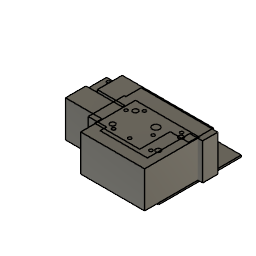
Valve mount (Autodesk Fusion 360 design; units mm, degrees)
Autodesk Fusion 360 part; units mm, degrees
sketch "Sketch3" plane through (0, 0, 0) normal (0, 0, 1) x (1, 0, 0)
  circle A0 centre (-19.4392, 58.0614) radius 3.5
  circle A1 centre (62.5608, 58.0614) radius 3.5
  circle A2 centre (-19.4392, -9.4386) radius 3.5
  circle A3 centre (62.5608, -9.4386) radius 3.5
  line L0 (-30, 76.3146) -> (73.519, 76.3146)
  line L1 (73.519, 76.3146) -> (73.519, -16.4944)
  line L2 (73.519, -16.4944) -> (-30, -16.4944)
  line L3 (-30, -16.4944) -> (-30, 76.3146)
  line L4 (73.519, 62.4381) -> (113.5114, 62.4381)
  line L5 (113.5114, 62.4381) -> (113.5114, -16.4944)
  line L6 (113.5114, -16.4944) -> (73.519, -16.4944)
  line L7 (73.519, -16.4944) -> (73.519, 62.4381)
  line L8 (-58.0351, -16.4944) -> (110, -16.4944)
  line L9 (110, -16.4944) -> (110, -50)
  line L10 (110, -50) -> (-58.0351, -50)
  line L11 (-58.0351, -50) -> (-58.0351, -16.4944)
  circle A4 centre (-250, -50) radius 5.5
  circle A5 centre (-250, 0) radius 5.5
  circle A6 centre (-150, -50) radius 5.5
  line L12 (-250, -50) -> (-250, 0) construction
  line L13 (-250, -50) -> (-150, -50) construction
  circle A7 centre (-150, 0) radius 5.5
  line L14 (-270, 20) -> (-130, 20)
  line L15 (-130, 20) -> (-130, -100)
  line L16 (-130, -100) -> (-270, -100)
  line L17 (-270, -100) -> (-270, 20)
  line L18 (-117.4884, 113.8078) -> (-158.4765, 113.8078) construction
  line L19 (-158.4765, 113.8078) -> (-152.4884, 113.8078) construction
  circle A8 centre (-117.4884, 113.8078) radius 3.5
  circle A9 centre (-152.4884, 113.8078) radius 3.5
  circle A10 centre (-174.4884, 162.8078) radius 3.5
  circle A11 centre (-97.4884, 145.3078) radius 3.5
  line L20 (-174.4884, 162.8078) -> (-87, 162.8078) construction
  line L21 (-97.4884, 145.3078) -> (-97.4884, 147.0826) construction
  line L22 (-97.4884, 147.0826) -> (-97.4884, 162.8078) construction
  line L23 (-117.4884, 113.8078) -> (-97.4884, 113.8078) construction
  line L24 (-97.4884, 113.8078) -> (-97.4884, 145.3078) construction
  line L25 (-184.4884, 103.8078) -> (-85.4884, 103.8078)
  line L26 (-85.4884, 103.8078) -> (-85.4884, 172.8078)
  line L27 (-85.4884, 172.8078) -> (-184.4884, 172.8078)
  line L28 (-184.4884, 172.8078) -> (-184.4884, 103.8078)
  line L29 (-184.4884, 120) -> (-264.4884, 120)
  line L30 (-264.4884, 120) -> (-264.4884, 165)
  line L31 (-264.4884, 165) -> (-184.4884, 165)
  line L32 (-184.4884, 165) -> (-184.4884, 120)
  line L33 (-44.9091, 170.4012) -> (-245, 170.4012)
  line L34 (-245, 170.4012) -> (-245, 225)
  line L35 (-245, 225) -> (-44.9091, 225)
  line L36 (-44.9091, 225) -> (-44.9091, 170.4012)
  circle A12 centre (-109.4884, 163.3078) radius 8
  dimension "d32" = 7
  dimension "d33" = 7
  dimension "d34" = 7
  dimension "d35" = 7
  dimension "d42" = 11
  dimension "d43" = 11
  dimension "d45" = 11
  dimension "d46" = 50
  dimension "d47" = 100
  dimension "d48" = 11
  dimension "d49" = 50
  dimension "d50" = 100
  dimension "d52" = 7
  dimension "d53" = 7
  dimension "d54" = 7
  dimension "d56" = 7
  dimension "d59" = 35
  dimension "d79" = 99
  dimension "d80" = 32
  dimension "d81" = 32
  dimension "d83" = 69
  dimension "d84" = 10
  dimension "d85" = 41.5
  dimension "d86" = 12
  dimension "d87" = 10
  dimension "d88" = 59
  dimension "d89" = 17.5
  dimension "d90" = 16
  dimension "d91" = 24
  dimension "d92" = 59.5
  constraint horizontal L0
  constraint vertical L1
  constraint horizontal L2
  constraint vertical L3
  constraint horizontal L4
  constraint vertical L5
  constraint horizontal L6
  constraint vertical L7
  constraint coincident L1 L4.start
  constraint horizontal L8
  constraint vertical L9
  constraint horizontal L10
  constraint vertical L11
  constraint coincident A4.centre L12.start
  constraint vertical L12
  constraint coincident A5.centre L12.end
  constraint perpendicular L12 L13
  constraint coincident A6.centre L13.end
  constraint horizontal L14
  constraint vertical L15
  constraint horizontal L16
  constraint vertical L17
  constraint perpendicular L17 L18
  constraint perpendicular L17 L19
  constraint coincident L18.start A8.centre
  constraint coincident L19.end A9.centre
  constraint coincident A10.centre L20.start
  constraint horizontal L20
  constraint coincident A11.centre L21.start
  constraint perpendicular L18 L21
  constraint coincident L20 L22.end
  constraint perpendicular L20 L22
  constraint perpendicular L21 L23
  constraint perpendicular L23 L24
  constraint horizontal L25
  constraint vertical L26
  constraint horizontal L27
  constraint vertical L28
  constraint horizontal L29
  constraint vertical L30
  constraint horizontal L31
  constraint vertical L32
  constraint coincident L28 L29.start
  constraint horizontal L33
  constraint vertical L34
  constraint horizontal L35
  constraint vertical L36
  measures "d32" diameter of A0
  measures "d33" diameter of A1
  measures "d34" diameter of A2
  measures "d35" diameter of A3
  measures "d42" diameter of A4
  measures "d43" diameter of A5
  measures "d45" diameter of A6
  measures "d46" distance of A4.centre A5.centre
  measures "d47" distance of A4.centre A6.centre
  measures "d48" diameter of A7
  measures "d49" distance of A6.centre A7.centre
  measures "d50" distance of A5.centre A7.centre
  measures "d52" diameter of A8
  measures "d53" diameter of A9
  measures "d54" diameter of A10
  measures "d56" diameter of A11
  measures "d59" distance of L18.start L19.end
  measures "d79" distance of L26 L28
  measures "d80" distance of L19.end L28
  measures "d81" distance of L18.start L26
  measures "d83" distance of L25.end L26.end
  measures "d84" distance of L18.start L25
  measures "d85" distance of A11.centre L25
  measures "d86" distance of A11.centre L26
  measures "d87" distance of A10.centre L28
  measures "d88" distance of A10.centre L25
  measures "d89" vertical distance of A10.centre A11.centre
  measures "d90" diameter of A12
  measures "d91" distance of L26 A12.centre
  measures "d92" distance of L25 A12.centre
extrude "Extrude2" add sketch "Sketch3" along normal blind 80 contours L0 L1 L2 L3 L7 L8 | L2 L6 L8 L9 L10 L11 | L1 L4 L5 L6 L7 L8 | L14 L15 L16 L17 | L25 L26 L28 L32 L33 A12 | L28 L29 L30 L31 L32 | L26 L27 L28 L33 A12 | L26 L27 L28 L33 L34 L35 L36 makes body 1 at (34.3722, 13.8549, 0) makes body 2 at (-215.5236, -84.7667, 0) makes body 3 at (-133.7259, 207.0357, 0)
extrude "Extrude3" add sketch "Sketch3" along normal blind -15 and the other way blind -5 contours A0 | A1 | A2 | A3 | A4 | A5 | A6 | A7 | A8 | A9 | A10 | A11 | L33 A12 | L33 A12 bodies 1 2 3
sketch "Sketch4" plane through (0, 0, 0) normal (0, 0, 1) x (1, 0, 0)
  line L0 (-60, -100) -> (235, -100)
  line L1 (235, -100) -> (235, -281)
  line L2 (-60, -190) -> (235, -190)
  line L3 (-60, -100) -> (-60, -190)
  line L4 (235, -281) -> (95, -281)
  line L5 (95, -281) -> (95, -190)
  dimension "d62" = 295
  dimension "d65" = 140
  dimension "d67" = 91
  dimension "d93" = 100
  dimension "d94" = 60
  dimension "d96" = 90
  constraint horizontal L0
  constraint vertical L1
  constraint coincident L1 L2.end
  constraint perpendicular L1 L2
  constraint perpendicular L1 L4
  constraint coincident L2 L5.end
  constraint perpendicular L2 L5
  measures "d62" distance of L0.start L0.end
  measures "d65" distance of L1.end L4.end
  measures "d67" distance of L4.end L5.end
  measures "d93" distance of origin L0
  measures "d94" horizontal distance of origin L0.start
  measures "d96" distance of L0 L2
extrude "Extrude4" add sketch "Sketch4" against normal blind 4 from surface at -2 separate body makes body 4
move_body "Move1" bodies 1 to x (1, 0, 0) y (0, 1, 0) z (0, 0, 1) at (-30, -175, 0)
move_body "Move2" bodies 2 to x (-1, 0, 0) y (0, -1, 0) z (0, 0, 1) at (-184.5, -172, 0)
move_body "Move3" bodies 3 to x (-1, 0, 0) y (0, -1, 0) z (0, 0, 1) at (-145.0248, -4.5371, -3.4865)
move_body "Move4" bodies 3 to x (1, 0, 0) y (0, 1, 0) z (0, 0, 1) at (25, 1, 3)
move_body "Move9" bodies 1 3 2 to x (1, 0, 0) y (0, 1, 0) z (0, 0, 1) at (0, 10, 0)
combine "Combine1" operation cut target body 4 tool bodies 3 2 1 keep tools
move_body "Move5" bodies 3 to x (1, 0, 0) y (0, 1, 0) z (0, 0, 1) at (170, 0, 0)
move_body "Move6" bodies 2 to x (1, 0, 0) y (0, 1, 0) z (0, 0, 1) at (150, 0, 0)
move_body "Move7" bodies 1 to x (1, 0, 0) y (0, 1, 0) z (0, 0, 1) at (170, 0, 0)
move_body "Move8" bodies 3 2 1 to x (-1, 0, 0) y (0, -1, 0) z (0, 0, 1) at (329.7685, -379.0742, 0)
move_body "Move10" bodies 2 to x (1, 0, 0) y (0, 1, 0) z (0, 0, 1) at (3, 3, 0)
combine "Combine3" operation cut target body 4 tool bodies 3 1 2 keep tools
sketch "ValveMount" plane through (0, 0, -6) normal (0, 0, -1) x (1, 0, 0)
  circle A0 centre (117.2685, 264.0742) radius 5.5
  circle A1 centre (217.2685, 264.0742) radius 5.5
  circle A2 centre (117.2685, 214.0742) radius 5.5
  circle A3 centre (217.2685, 214.0742) radius 5.5
  circle A4 centre (209.2077, 204.6356) radius 3.5
  circle A5 centre (127.2077, 204.6356) radius 3.5
  circle A6 centre (182.3049, 240.2293) radius 3.5
  circle A7 centre (105.3049, 222.7293) radius 3.5
  circle A8 centre (-49.4392, 174.4386) radius 3.5
  circle A9 centre (32.5608, 174.4386) radius 3.5
  circle A10 centre (-49.4392, 106.9386) radius 3.5
  circle A11 centre (65.5, 112) radius 5.5
  circle A12 centre (-34.5, 112) radius 5.5
  circle A13 centre (65.5, 162) radius 5.5
  circle A14 centre (-34.5, 162) radius 5.5
  circle A15 centre (-2.5364, 107.3449) radius 3.5
  circle A16 centre (-22.5364, 138.8449) radius 3.5
  circle A17 centre (54.4636, 156.3449) radius 3.5
  line L0 (-60, 190) -> (-60, 100)
  line L1 (-60, 100) -> (235, 100)
  line L2 (235, 100) -> (235, 281)
  line L3 (235, 281) -> (95, 281)
  line L4 (95, 281) -> (95, 190)
  line L5 (95, 190) -> (-60, 190)
  circle A18 centre (117.2685, 264.0742) radius 5.5
  circle A19 centre (217.2685, 264.0742) radius 5.5
  circle A20 centre (117.2685, 214.0742) radius 5.5
  circle A21 centre (217.2685, 214.0742) radius 5.5
  circle A22 centre (209.2077, 204.6356) radius 3.5
  circle A23 centre (127.2077, 204.6356) radius 3.5
  circle A24 centre (182.3049, 240.2293) radius 3.5
  circle A25 centre (105.3049, 222.7293) radius 3.5
  circle A26 centre (-49.4392, 174.4386) radius 3.5
  circle A27 centre (32.5608, 174.4386) radius 3.5
  circle A28 centre (-49.4392, 106.9386) radius 3.5
  circle A29 centre (65.5, 112) radius 5.5
  circle A30 centre (-34.5, 112) radius 5.5
  circle A31 centre (65.5, 162) radius 5.5
  circle A32 centre (-34.5, 162) radius 5.5
  circle A33 centre (-2.5364, 107.3449) radius 3.5
  circle A34 centre (-22.5364, 138.8449) radius 3.5
  circle A35 centre (54.4636, 156.3449) radius 3.5
  line L6 (-60, 190) -> (95, 190)
  line L7 (95, 281) -> (95, 190)
  line L8 (235, 281) -> (95, 281)
  line L9 (235, 100) -> (235, 281)
  line L10 (-60, 100) -> (235, 100)
  line L11 (-60, 100) -> (-60, 190)
  line L12 (95, 190) -> (95, 100)
  circle A36 centre (-10.5364, 156.8449) radius 8
  arc A37 (29.1144, 106.3286) -> (35.91, 107.9549) centre (32.5608, 106.9386) ccw
  arc A38 (35.91, 107.9549) -> (29.1144, 106.3286) centre (32.4636, 107.3449) ccw
  arc A39 (123.8585, 271.1193) -> (130.6541, 272.7456) centre (127.3049, 271.7293) ccw
  circle A40 centre (170.3049, 222.2293) radius 8
  arc A41 (123.8585, 271.1193) -> (130.6541, 272.7456) centre (127.3049, 271.7293) ccw
  circle A42 centre (170.3049, 222.2293) radius 8
  arc A43 (29.1144, 106.3286) -> (35.91, 107.9549) centre (32.5608, 106.9386) ccw
  arc A44 (35.91, 107.9549) -> (29.1144, 106.3286) centre (32.4636, 107.3449) ccw
  circle A45 centre (-10.5364, 156.8449) radius 8
  circle A46 centre (162.3049, 271.7293) radius 3.5
  arc A47 (130.6541, 272.7456) -> (123.8585, 271.1193) centre (127.2077, 272.1356) ccw
  circle A48 centre (209.2077, 272.1356) radius 3.5
  circle A49 centre (209.2077, 272.1356) radius 3.5
  arc A50 (130.6541, 272.7456) -> (123.8585, 271.1193) centre (127.2077, 272.1356) ccw
  circle A51 centre (162.3049, 271.7293) radius 3.5
  dimension "d71" = 140
  dimension "d72" = 155
  dimension "d73" = 90
  dimension "d74" = 91
  constraint coincident L4.end L5.start
  constraint coincident L10 L12.end
  constraint perpendicular L10 L12
  measures "d72" distance of L0.start L4.end
  measures "d73" distance of L0.start L0.end
extrude "Extrude5" add sketch "ValveMount" along normal blind 2 separate body contours L0 L1 L5 L6 L10 L11 L12 makes body 5
equation "ValveMount_Short = 50 mm" comment "Valve Mount M10 hole Short side"
equation "ValveMount_Long = 100 mm" comment "Valve Mount M10 hole Short side"
named bodies: "baraki_OC", "hektos_OC", "baraki_LS", "plate"
